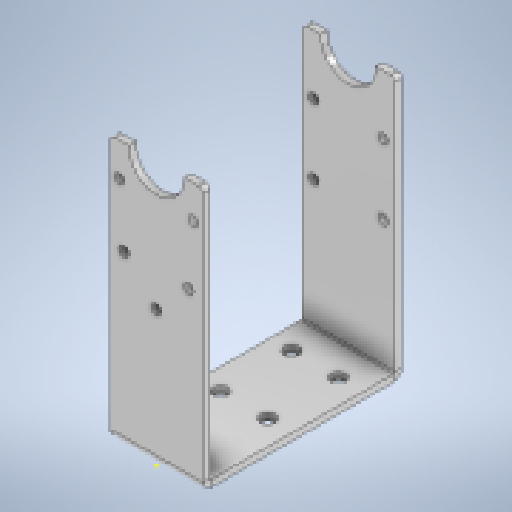
# Autodesk Inventor part: axis_16_top_frame
Saved by Autodesk Inventor 2026.1 (Build 301233000, 233)
## iProperties
Created: 2025-06-30
Part Number: axis_16_top_frame
Material: Aluminum 6061-AHC
Document SubType Name: Sheet Metal
Designer: LG
Density: 2.7 g/cm^3
Sheet Metal Rule: Default_mm
Appearance: Aluminum - Dark
Flat Pattern Width: 2.014 cm
Flat Pattern Length: 15.1659 cm
Flat Pattern Area: 30.544 cm^2
Sheet Metal Width: 20.140 mm
Sheet Metal Length: 151.659 mm
Sheet Metal Area: 3054.403 mm^2
Author: LG
Autodesk Inventor part; units mm, degrees
ref_plane "YZ Plane" through (0, 0, 0) normal (1, 0, 0) x (0, 1, 0)
ref_plane "XZ Plane" through (0, 0, 0) normal (0, 1, 0) x (-1, 0, 0)
ref_plane "XY Plane" through (0, 0, 0) normal (0, 0, 1) x (1, 0, 0)
sketch "Sketch1" plane through (0, 0, 0) normal (0, 1, 0) x (-1, 0, 0)
  line L0 (10.07, 20.05) -> (-10.07, 20.05)
  line L1 (-10.07, 20.05) -> (-10.07, -20.05)
  line L2 (-10.07, -20.05) -> (10.07, -20.05)
  line L3 (10.07, -20.05) -> (10.07, 20.05)
  point P0 (0, 0)
  dimension "d0" = 40.1
  dimension "d1" = 20.14
  dimension "d2" = 10.07
  dimension "d3" = 20.05
  measures "d0" distance of L2.end L0.start
  measures "d1" distance of L1.end L2.end
  measures "d2" distance from line of point (0, 0) L3
  measures "d3" distance from line of point (0, 0) L2
extrude "Plate1" add sketch "Sketch1" along normal blind 1.5
sketch "Sketch2" plane through (10.07, 0, 21.55) normal (0, 0, -1) x (-1, 0, 0)
  line L0 (20.14, 0) -> (0, 0)
  line L1 (0, 0) -> (0, 57)
  line L2 (0, 57) -> (20.14, 57)
  line L3 (20.14, 57) -> (20.14, 0)
  constraints: 8 end point
edge flange "Flange1" height 57 angle 90 thickness 1.5 bend radius 0.31 thickness toward (0, 0, -1) relief straight relief width 1.5 relief depth 0.75 corner gap 0.31 corner form 0 edges at (0, 1.5, 20.05) (0, 1.5, -20.05) wall of the first edge with corners at (-10.07, 0, 21.55) (10.07, 0, 21.55) (10.07, 57, 21.55) (-10.07, 57, 21.55)
bend "Bend1"
corner "Corner1"
sketch "Sketch15" plane through (10.07, 57, -21.55) normal (0, 0, -1) x (-1, 0, 0)
  circle A0 centre (2.545, -12.76) radius 0.7835
  circle A1 centre (17.595, -12.76) radius 0.7835
  circle A2 centre (2.545, -27.86) radius 0.7835
  circle A3 centre (17.595, -27.86) radius 0.7835
  point P0 (10.07, -57)
  constraints: 4 centre point, 8 other
hole "Hole9" at (7.525, 44.24, -21.55) at (-7.525, 44.24, -21.55) at (7.525, 29.14, -21.55) at (-7.525, 29.14, -21.55) direction (0, 0, 1) diameter 2.1 depth 1.5
sketch "Sketch16" plane through (-10.07, 57, 21.55) normal (0, 0, 1) x (1, 0, 0)
  circle A0 centre (18.07, -7.16) radius 0.7835
  circle A1 centre (2.07, -7.16) radius 0.7835
  circle A2 centre (3.07, -20.38) radius 0.7835
  circle A3 centre (17.07, -20.38) radius 0.7835
  circle A4 centre (10.07, -27.68) radius 0.7835
  point P0 (10.07, -57)
  constraints: 5 centre point, 10 other
hole "Hole10" at (-8, 49.84, 21.55) at (8, 49.84, 21.55) at (-7, 36.62, 21.55) at (7, 36.62, 21.55) at (0, 29.32, 21.55) direction (0, 0, -1) diameter 2.1 depth 1.5
sketch "Sketch17" plane through (-10.07, 57, 21.55) normal (0, 0, 1) x (1, 0, 0)
  point P0 (10.07, -57)
sketch "Sketch18" plane through (-10.07, 57, 21.55) normal (0, 0, 1) x (1, 0, 0)
  point P0 (10.07, -57)
sketch "Sketch19" plane through (-10.07, 57, 21.55) normal (0, 0, 1) x (1, 0, 0)
  circle A0 centre (10.07, -0.26) radius 6
  point P0 (10.07, -57)
  constraints: 1 centre point, 2 other
extrude "Cut5" cut sketch "Sketch19" against normal blind 1.5
sketch "Sketch20" plane through (10.07, 57, -21.55) normal (0, 0, -1) x (-1, 0, 0)
  circle A0 centre (10.07, -0.26) radius 6
  point P0 (10.07, -57)
  constraints: 1 centre point, 2 other
extrude "Cut6" cut sketch "Sketch20" against normal blind 1.5
fillet "Corner Round1" radius 1 4 edges at (10.07, 57, 20.8) (10.07, 57, -20.8) (-10.07, 57, -20.8) (-10.07, 57, 20.8)
sketch "Sketch22" plane through (0, 1.5, 0) normal (0, 1, 0) x (1, 0, 0)
  point P0 (0, 0)
sketch "Sketch23" plane through (0, 1.5, 0) normal (0, 1, 0) x (1, 0, 0)
  point P0 (0, 0)
sketch "Sketch24" plane through (0, 1.5, 0) normal (0, 1, 0) x (1, 0, 0)
  circle A0 centre (4.76, -13.05) radius 1.55 projected
  circle A1 centre (-5.38, -13.05) radius 1.55 projected
  circle A2 centre (-5.38, 2.25) radius 1.55 projected
  circle A3 centre (4.76, 2.25) radius 1.55 projected
  point P0 (0, 0)
hole "Hole12" at (4.76, 1.5, 13.05) at (-5.38, 1.5, 13.05) at (4.76, 1.5, -2.25) at (-5.38, 1.5, -2.25) direction (0, -1, 0) diameter 3.1 end through all
equation "\"d96\" = Thickness"
equation "\"d103\" = Thickness"
equation "\"d105\" = Thickness"
equation "\"d107\" = Thickness"
equation "\"d124\" = Thickness"
equation "\"d4\" = Thickness"
equation "\"d5\" = BendReliefWidth"
equation "\"d6\" = BendReliefDepth"
equation "\"d7\" = MinimumRemnant"
equation "\"d8\" = TransitionRadius"
equation "\"d11\" = BendRadius"
equation "\"d12\" = CornerReliefSize"
equation "\"d13\" = GapSize"
equation "\"d14\" = JacobiRadiusSize"
equation "\"BendReliefWidth\" = Thickness"
equation "\"BendReliefDepth\" = 0.5 * Thickness"
equation "\"CornerReliefSize\" = 4 * Thickness"
equation "\"MinimumRemnant\" = 2 * Thickness"
equation "\"TransitionRadius\" = BendRadius"
equation "\"JacobiRadiusSize\" = BendRadius"
equation "\"GapSize\" = Thickness"
equation "\"Thickness\" = 1.5"
equation "\"BendRadius\" = 0.31"
body "Solid1"
